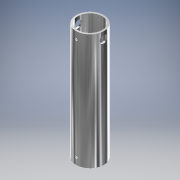
# Autodesk Inventor part: rura_30_2_250
Saved by Autodesk Inventor 2017 (Build 210142000, 142)
## iProperties
Created: 2017-03-22
Part Number: rura_30_2_250
Material: Aluminium 6061
Document SubType Name: Modeling
Designer: Damian
Density: 2.7 g/cm^3
Appearance: Aluminium — płaski
Mass: 114.622 g
Surface Area: 433.282 cm^2
Volume: 42.4527 cm^3
Author: Damian
Autodesk Inventor part; units mm, degrees
ref_plane "YZ Plane" through (0, 0, 0) normal (1, 0, 0) x (0, 1, 0)
ref_plane "XZ Plane" through (0, 0, 0) normal (0, 1, 0) x (-1, 0, 0)
ref_plane "XY Plane" through (0, 0, 0) normal (0, 0, 1) x (1, 0, 0)
sketch "Szkic1" plane through (0, 0, 0) normal (0, 0, 1) x (1, 0, 0)
  circle A0 centre (0, 0) radius 15
  circle A1 centre (0, 0) radius 13
  dimension "d0" = 30
  dimension "d2" = 2
  constraints: 3 coincident, 2 centre point
  measures "d0" diameter of A0
  measures "d2" radial gap between concentric circles of A1 A0
extrude "Wyciągnięcie proste1" add sketch "Szkic1" along normal mid plane 125
sketch "Szkic5" plane through (0, 0, 0) normal (0, 1, 0) x (-1, 0, 0)
  circle A0 centre (0, 55) radius 1.5
  circle A1 centre (0, -55) radius 1.5
  point P0 (0, 0)
  dimension "d40" = 3
  dimension "d41" = 3
  constraints: 2 centre point
  measures "d40" diameter of A0
  measures "d41" diameter of A1
extrude "Wyciągnięcie proste6" cut sketch "Szkic5" against normal blind 20
sketch "Szkic6" plane through (0, 0, 0) normal (1, 0, 0) x (0, 1, 0)
  circle A0 centre (0, 55) radius 4
  point P0 (0, 0)
  dimension "d44" = 8
  constraints: 1 centre point
  measures "d44" diameter of A0
extrude "Wyciągnięcie proste7" cut sketch "Szkic6" along normal mid plane 30
